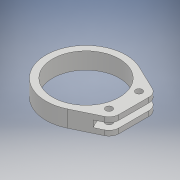
# Autodesk Inventor part: double spring swivel 6
Saved by Autodesk Inventor 2017 (Build 210142000, 142)
## iProperties
Created: 2018-07-24
Part Number: double spring swivel 6
Material: Generic
Document SubType Name: Modeling
Designer: jakub.tomczynski
Density: 1 g/cm^3
Appearance: Default
Author: jakub.tomczynski
Autodesk Inventor part; units mm, degrees
ref_plane "YZ Plane" through (0, 0, 0) normal (1, 0, 0) x (0, 1, 0)
ref_plane "XZ Plane" through (0, 0, 0) normal (0, 1, 0) x (-1, 0, 0)
ref_plane "XY Plane" through (0, 0, 0) normal (0, 0, 1) x (1, 0, 0)
sketch "Sketch1" plane through (0, 0, 0) normal (0, 0, 1) x (1, 0, 0)
  circle A0 centre (0, 0) radius 5
  circle A1 centre (5.7, 2.25) radius 0.5
  circle A2 centre (5.7, -2.25) radius 0.5
  line L0 (0, 0) -> (12.1327, 0) construction
  arc A3 (7.2, 2.25) -> (6.3507, 3.6015) centre (5.7, 2.25) ccw
  arc A4 (6.3507, -3.6015) -> (7.2, -2.25) centre (5.7, -2.25) ccw
  line L1 (2.6029, 5.406) -> (6.3507, 3.6015)
  line L2 (2.6029, -5.406) -> (6.3507, -3.6015)
  line L3 (7.2, -2.25) -> (7.2, 2.25)
  arc A5 (2.6029, 5.406) -> (2.6029, -5.406) centre (0, 0) ccw
  dimension "d1" = 10
  dimension "d12" = 1
  dimension "d13" = 1
  dimension "d14" = 4.5
  dimension "d16" = 3
  dimension "d17" = 3
  dimension "d18" = 5.7
  dimension "d19" = 6
  constraints: 8 end point, 7 point on circle, 6 centre point, 6 tangent, 4 coincident, 1 horizontal, 1 point on line, 1 symmetric about line
  measures "d1" diameter of A0
  measures "d12" diameter of A1
  measures "d13" diameter of A2
  measures "d14" distance of A2.centre A1.centre
  measures "d16" diameter of A3
  measures "d17" diameter of A4
  measures "d18" horizontal distance of A1.centre point (0, 0)
  measures "d19" radius of A5
extrude "Extrusion1" add sketch "Sketch1" along normal mid plane 2.5
sketch "Sketch2" plane through (0, 0, 0) normal (0, 0, 1) x (1, 0, 0)
  circle A0 centre (5.7, 2.25) radius 0.5 projected
  circle A1 centre (5.7, -2.25) radius 0.5 projected
  line L0 (7.65, 2.25) -> (7.65, -2.25) construction
  line L1 (4.6, 2.25) -> (4.6, -2.25)
  line L2 (10.7, -2.25) -> (10.7, 2.25)
  arc A2 (10.7, 2.25) -> (4.6, 2.25) centre (7.65, 2.25) ccw
  arc A3 (4.6, -2.25) -> (10.7, -2.25) centre (7.65, -2.25) ccw
  point P0 (0, 0)
  point P1 (7.65, 0)
  dimension "d20" = 1.1
  dimension "d21" = 5
  constraints: 8 end point, 4 point on circle, 4 tangent, 2 centre point, 2 horizontal alignment, 1 midpoint, 1 parallel, 1 vertical
  measures "d20" distance from line of A0.centre L1
  measures "d21" distance from line of L2 A0.centre
extrude "Extrusion2" cut sketch "Sketch2" along normal mid plane 1
body "Solid1"
